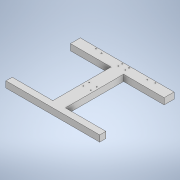
# Autodesk Inventor part: 固定架
Saved by Autodesk Inventor 2020 (Build 240168000, 168)
## iProperties
Created: 2020-12-03
Part Number: 固定架
Material: 常规
Document SubType Name: Sheet Metal
Designer: huang
Density: 1 g/cm^3
Sheet Metal Rule: 默认_mm
Appearance: 默认
Author: huang
Autodesk Inventor part; units mm, degrees
ref_plane "YZ Plane" through (0, 0, 0) normal (1, 0, 0) x (0, 1, 0)
ref_plane "XZ Plane" through (0, 0, 0) normal (0, 1, 0) x (-1, 0, 0)
ref_plane "XY Plane" through (0, 0, 0) normal (0, 0, 1) x (1, 0, 0)
sketch "草图1" plane through (0, 0, 0) normal (0, 1, 0) x (-1, 0, 0)
  line L0 (16.7619, 206.381) -> (-23.2381, 206.381)
  line L1 (-23.2381, 206.381) -> (-23.2381, -31.619)
  line L2 (-23.2381, -31.619) -> (16.7619, -31.619)
  line L3 (16.7619, -31.619) -> (16.7619, 206.381)
  point P0 (0, 0)
  dimension "d0" = 40
  dimension "d1" = 238
  constraints: 8 end point, 2 parallel, 1 horizontal, 1 perpendicular
  measures "d0" distance of L1.end L2.end
  measures "d1" distance of L2.end L0.start
extrude "拉伸1" add sketch "草图1" along normal blind 20
sketch "草图2" plane through (23.2381, 0, 206.381) normal (1, 0, 0) x (0, 0, -1)
  line L0 (238, 20) -> (0, 20) projected
  line L1 (238, 0) -> (0, 0) projected
  line L2 (0, 20) -> (20, 20)
  line L3 (20, 20) -> (20, 0)
  line L4 (20, 0) -> (0, 0)
  line L5 (0, 0) -> (0, 20)
  point P0 (206.381, 0)
  dimension "d4" = 20
  constraints: 8 end point, 2 parallel, 1 horizontal, 1 perpendicular, 1 point on line
  measures "d4" distance between parallel lines of L3 L5
extrude "拉伸2" add sketch "草图2" along normal blind 20
sketch "草图5" plane through (-16.7619, 0, -31.619) normal (-1, 0, 0) x (0, 0, 1)
  line L0 (0, 0) -> (238, 0) projected
  line L1 (218, 20) -> (0, 20) projected
  line L2 (238, 0) -> (218, 0)
  line L3 (218, 0) -> (218, 20)
  line L4 (218, 20) -> (238, 20)
  line L5 (238, 20) -> (238, 0)
  point P0 (31.619, 0)
  constraints: 8 end point, 2 parallel, 1 horizontal, 1 perpendicular
extrude "拉伸3" add sketch "草图5" along normal blind 20
sketch "草图6" plane through (-16.7619, 0, -31.619) normal (-1, 0, 0) x (0, 0, 1)
  line L0 (0, 0) -> (0, 20) projected
  line L1 (218, 0) -> (0, 0) projected
  line L2 (0, 20) -> (20, 20)
  line L3 (20, 20) -> (20, 0)
  line L4 (20, 0) -> (0, 0)
  line L5 (0, 0) -> (0, 20)
  point P0 (31.619, 0)
  dimension "d9" = 20
  constraints: 8 end point, 2 parallel, 1 horizontal, 1 perpendicular, 1 point on line
  measures "d9" distance between parallel lines of L3 L0
extrude "拉伸4" add sketch "草图6" along normal blind 20
sketch "草图7" plane through (23.2381, 0, -31.619) normal (1, 0, 0) x (0, 0, -1)
  line L0 (0, 0) -> (0, 20) projected
  line L1 (-20, 0) -> (-218, 0) projected
  line L2 (0, 20) -> (-20, 20)
  line L3 (-20, 20) -> (-20, 0)
  line L4 (-20, 0) -> (0, 0)
  line L5 (0, 0) -> (0, 20)
  point P0 (-31.619, 0)
  constraints: 8 end point, 2 parallel, 1 horizontal, 1 perpendicular
extrude "拉伸5" add sketch "草图7" along normal blind 20
sketch "草图8" plane through (0, 20, 0) normal (0, 1, 0) x (1, 0, 0)
  line L0 (23.2381, -186.381) -> (23.2381, 11.619) projected
  line L1 (-16.7619, 11.619) -> (-16.7619, -186.381) projected
  circle A0 centre (-8.7619, -96.881) radius 1.5
  circle A1 centre (-8.7619, -77.881) radius 1.5
  circle A2 centre (15.2381, -96.881) radius 1.5
  circle A3 centre (15.2381, -77.881) radius 1.5
  point P0 (0, 0)
  constraints: 4 centre point
extrude "拉伸6" cut sketch "草图8" against normal through all
sketch "草图9" plane through (0, 20, 0) normal (0, 1, 0) x (1, 0, 0)
  line L0 (-36.7619, 31.619) -> (43.2381, 31.619) projected
  line L1 (3.2381, 31.619) -> (3.2381, -247.5925)
  line L2 (3.2381, 31.619) -> (153.2381, 31.619)
  line L3 (3.2381, 31.619) -> (-146.7619, 31.619)
  line L4 (-146.7619, 31.619) -> (-146.7619, 11.619)
  line L5 (-16.7619, 11.619) -> (-36.7619, 11.619) projected
  line L6 (-146.7619, 11.619) -> (153.2381, 11.619)
  line L7 (153.2381, 11.619) -> (153.2381, 31.619)
  line L8 (-146.7619, -186.381) -> (153.2381, -186.381)
  line L9 (153.2381, -186.381) -> (153.2381, -206.381)
  line L10 (43.2381, -206.381) -> (-36.7619, -206.381) projected
  line L11 (153.2381, -206.381) -> (-146.7619, -206.381)
  line L12 (-146.7619, -206.381) -> (-146.7619, -186.381)
  point P0 (0, 0)
  dimension "d20" = 150
  dimension "d21" = 150
  constraints: 20 end point, 6 perpendicular, 3 horizontal, 1 midpoint, 1 vertical
  measures "d20" distance of L1.start L2.end
  measures "d21" distance of L1.start L3.end
extrude "拉伸7" add sketch "草图9" against normal blind 20
sketch "草图10" plane through (0, 20, 0) normal (0, 1, 0) x (1, 0, 0)
  line L0 (3.2381, 42.6) -> (3.2381, -82.4296)
  line L1 (-146.7619, 31.619) -> (153.2381, 31.619) projected
  line L2 (3.2381, 31.619) -> (3.2381, 26.619)
  line L3 (3.2381, 26.619) -> (14.2381, 26.619)
  line L4 (14.2381, 26.619) -> (-7.7619, 26.619)
  circle A0 centre (-7.7619, 26.619) radius 1.5
  circle A1 centre (14.2381, 26.619) radius 1.5
  line L5 (14.2381, 26.619) -> (14.2381, 14.619)
  circle A2 centre (14.2381, 14.619) radius 1.5
  line L6 (-7.7619, 26.619) -> (-7.7619, 14.619)
  circle A3 centre (-7.7619, 14.619) radius 1.5
  point P0 (0, 0)
  dimension "d27" = 5
  dimension "d28" = 11
  dimension "d29" = 22
  dimension "d30" = 3
  dimension "d31" = 3
  dimension "d32" = 12
  dimension "d33" = 3
  dimension "d34" = 12
  dimension "d35" = 3
  constraints: 12 end point, 4 centre point, 4 coincident, 3 vertical, 2 point on line, 1 midpoint, 1 perpendicular
  measures "d27" distance of L2.start L2.end
  measures "d28" distance of L2.end L3.end
  measures "d29" distance of L3.end L4.end
  measures "d30" diameter of A0
  measures "d31" diameter of A1
  measures "d32" distance of L5.start L5.end
  measures "d33" diameter of A2
  measures "d34" distance of L6.start L6.end
  measures "d35" diameter of A3
extrude "拉伸8" cut sketch "草图10" against normal through all
sketch "草图12" plane through (0, 20, 0) normal (0, 1, 0) x (1, 0, 0)
  line L0 (-146.7619, 31.619) -> (-91.7619, 31.619)
  line L1 (-91.7619, 31.619) -> (-91.7619, 26.619)
  circle A0 centre (-91.7619, 26.619) radius 1.5
  line L2 (3.2381, 31.619) -> (3.2381, -27.4763)
  line L3 (98.2381, 31.619) -> (98.2381, 26.619)
  circle A1 centre (98.2381, 26.619) radius 1.5
  line L4 (-91.7619, 26.619) -> (-70.0961, 22.7988)
  circle A2 centre (14.2381, 26.619) radius 1.5 projected
  circle A3 centre (-7.7619, 26.619) radius 1.5 projected
  circle A4 centre (-70.0961, 22.7988) radius 1.5
  circle A5 centre (76.5723, 22.7988) radius 1.5
  point P0 (0, 0)
  dimension "d43" = 55
  dimension "d50" = 22
  dimension "d51" = 3
  dimension "d58" = 100
  dimension "d59" = 5
  constraints: 10 end point, 4 centre point, 4 symmetric about line, 3 coincident, 1 perpendicular, 1 vertical, 2 other
  measures "d43" distance of L0.start L0.end
  measures "d50" distance of L4.start L4.end
  measures "d51" diameter of A4
  measures "d58" angle of L4 L1
  measures "d59" distance of L0.end L1.end
extrude "拉伸9" cut sketch "草图12" against normal through all contours A0 L4 L1 | A4 | L1 L4 A0 | A1 | A5
sketch "草图13" plane through (23.2381, 0, 186.381) normal (1, 0, 0) x (0, 0, -1)
  line L0 (0, 20) -> (198, 20) projected
  line L1 (198, 20) -> (186.381, 20)
  line L2 (186.381, 20) -> (186.381, 0)
  line L3 (186.381, 0) -> (198, 0)
  line L4 (198, 0) -> (198, 20)
  constraints: 8 end point, 2 parallel, 1 horizontal, 1 perpendicular
extrude "拉伸10" add sketch "草图13" along normal blind 130 and the other way blind 5
sketch "草图14" plane through (-16.7619, 0, 186.381) normal (-1, 0, 0) x (0, 0, 1)
  line L0 (-198, 20) -> (-198, 0) projected
  line L1 (-186.381, 0) -> (-186.381, 20) projected
  line L2 (-198, 0) -> (-186.381, 0)
  line L3 (-186.381, 0) -> (-186.381, 20)
  line L4 (-186.381, 20) -> (-198, 20)
  line L5 (-198, 20) -> (-198, 0)
  point P0 (-197.5, 20)
  constraints: 8 end point, 2 parallel, 1 horizontal, 1 perpendicular
extrude "拉伸11" add sketch "草图14" along normal blind 130
equation "\"折弯半径\" = 厚度"
equation "\"折弯释压宽度\" = 厚度"
equation "\"折弯释压深度\" = 0.5 * 厚度"
equation "\"拐角释压尺寸\" = 4 * 厚度"
equation "\"最小余量\" = 2 * 厚度"
equation "\"过渡半径\" = 折弯半径"
equation "\"Jacobi半径尺寸\" = 折弯半径"
equation "\"间隙大小\" = 厚度"
equation "\"厚度\" = 0.5"
